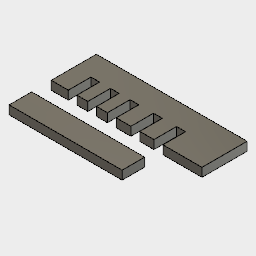
test kit with dog bone (Autodesk Fusion 360 design; units mm, degrees)
Autodesk Fusion 360 part; units mm, degrees
note: some values were not read from the file. Set by a fixed rule: which sketch regions a step uses.
sketch "Sketch1" plane through (0, 0, 0) normal (0, 1, 0) x (1, 0, 0)
  line L0 (-84.8022, -30) -> (-72.2022, -30)
  line L1 (-72.2022, -30) -> (-72.2022, 0)
  line L2 (-72.2022, 0) -> (-84.8022, 0)
  line L3 (-84.8022, 0) -> (-84.8022, -30)
  line L4 (-53.694, -30) -> (-40.994, -30)
  line L5 (-40.994, -30) -> (-40.994, 0)
  line L6 (-40.994, 0) -> (-53.694, 0)
  line L7 (-53.694, 0) -> (-53.694, -30)
  line L8 (-23.1582, -30) -> (-10.3582, -30)
  line L9 (-10.3582, -30) -> (-10.3582, 0)
  line L10 (-10.3582, 0) -> (-23.1582, 0)
  line L11 (-23.1582, 0) -> (-23.1582, -30)
  line L12 (-99.2349, -30) -> (-111.7349, -30)
  line L13 (-111.7349, -30) -> (-111.7349, 0)
  line L14 (-111.7349, 0) -> (-99.2349, 0)
  line L15 (-99.2349, 0) -> (-99.2349, -30)
  line L16 (-125.224, -30) -> (-137.624, -30)
  line L17 (-137.624, -30) -> (-137.624, 0)
  line L18 (-137.624, 0) -> (-125.224, 0)
  line L19 (-125.224, 0) -> (-125.224, -30)
  line L20 (-159.4563, -30) -> (40.5437, -30)
  line L21 (40.5437, -30) -> (40.5437, 30)
  line L22 (40.5437, 30) -> (-159.4563, 30)
  line L23 (-159.4563, 30) -> (-159.4563, -30)
  dimension "d3" = 12.6
  dimension "d4" = 30
  dimension "d6" = 12.7
  dimension "d7" = 30
  dimension "d8" = 12.8
  dimension "d9" = 30
  dimension "d10" = 12.5
  dimension "d11" = 30
  dimension "d12" = 12.4
  dimension "d13" = 30
  dimension "d14" = 200
  dimension "d15" = 60
  measures "d3" distance of L0.start L0.end
  measures "d4" distance of L0.start L2.end
  measures "d6" distance of L4.start L4.end
  measures "d7" distance of L4.start L6.end
  measures "d8" distance of L8.start L8.end
  measures "d9" distance of L8.start L10.end
  measures "d10" distance of L12.start L12.end
  measures "d11" distance of L12.start L14.end
  measures "d12" distance of L16.start L16.end
  measures "d13" distance of L16.start L18.end
  measures "d14" distance of L20.start L20.end
  measures "d15" distance of L20.start L22.end
extrude "Extrude1" add sketch "Sketch1" along normal blind 11.6 contours L1 L2 L3 L5 L6 L7 L9 L10 L11 L13 L14 L15 L17 L18 L19 L20 L21 L22 L23 makes body 1
sketch "Sketch2" plane through (0, 11.6, 0) normal (0, 1, 0) x (-1, 0, 0)
  line L0 (10.3582, 30) -> (-40.5437, 30)
  line L1 (-40.5437, 30) -> (-40.5437, -30)
  line L2 (-40.5437, -30) -> (159.4563, -30)
  line L3 (159.4563, -30) -> (159.4563, 30)
  line L4 (159.4563, 30) -> (137.624, 30)
  line L5 (137.624, 30) -> (137.624, 0)
  line L6 (137.624, 0) -> (125.224, 0)
  line L7 (125.224, 0) -> (125.224, 30)
  line L8 (125.224, 30) -> (111.7349, 30)
  line L9 (111.7349, 30) -> (111.7349, 0)
  line L10 (111.7349, 0) -> (99.2349, 0)
  line L11 (99.2349, 0) -> (99.2349, 30)
  line L12 (99.2349, 30) -> (84.8022, 30)
  line L13 (84.8022, 30) -> (84.8022, 0)
  line L14 (84.8022, 0) -> (72.2022, 0)
  line L15 (72.2022, 0) -> (72.2022, 30)
  line L16 (72.2022, 30) -> (53.694, 30)
  line L17 (53.694, 30) -> (53.694, 0)
  line L18 (53.694, 0) -> (40.994, 0)
  line L19 (40.994, 0) -> (40.994, 30)
  line L20 (40.994, 30) -> (23.1582, 30)
  line L21 (23.1582, 30) -> (23.1582, 0)
  line L22 (23.1582, 0) -> (10.3582, 0)
  line L23 (10.3582, 0) -> (10.3582, 30)
  line L24 (159.1299, 46.1552) -> (9.1299, 46.1552)
  line L25 (9.1299, 46.1552) -> (9.1299, 76.1552)
  line L26 (9.1299, 76.1552) -> (159.1299, 76.1552)
  line L27 (159.1299, 76.1552) -> (159.1299, 46.1552)
  dimension "d18" = 150
  dimension "d19" = 30
  measures "d18" distance of L24.start L24.end
  measures "d19" distance of L24.start L26.end
extrude "Extrude2" add sketch "Sketch2" along normal blind 11.6 separate body contours L24 L25 L26 L27 makes body 2
move_body "Move1" bodies 2 to x (1, 0, 0) y (0, 1, 0) z (0, 0, 1) at (0, 0, 10)
move_body "Align1" bodies 2 to x (1, 0, 0) y (0, 1, 0) z (0, 0, 1) at (0, -11.6, 0)
sketch "Sketch3" plane through (0, 0, 0) normal (0, 1, 0) x (1, 0, 0)
  line L0 (-135.0903, -41.1348) -> (-85.0903, -41.1348)
  line L1 (-85.0903, -41.1348) -> (-85.0903, -68.6348)
  line L2 (-85.0903, -68.6348) -> (-135.0903, -68.6348)
  line L3 (-135.0903, -68.6348) -> (-135.0903, -41.1348)
  dimension "d22" = 50
  dimension "d23" = 27.5
  measures "d22" distance of L0.start L0.end
  measures "d23" distance of L0.start L2.end
extrude "Extrude3" add sketch "Sketch3" along normal blind 11.6 separate body makes body 3
delete_body "RemoveBody1" bodies 2
move_body "Move2" bodies 3 to x (1, 0, 0) y (0, 1, 0) z (0, 0, 1) at (-20, 0, 20)
sketch "Sketch4" plane through (0, 11.6, 0) normal (0, 1, 0) x (-1, 0, 0)
  line L0 (10.3582, 30) -> (-40.5437, 30)
  line L1 (-40.5437, 30) -> (-40.5437, -30)
  line L2 (-40.5437, -30) -> (159.4563, -30)
  line L3 (159.4563, -30) -> (159.4563, 30)
  line L4 (159.4563, 30) -> (137.624, 30)
  line L5 (137.624, 30) -> (137.624, 0)
  line L6 (137.624, 0) -> (125.224, 0)
  line L7 (125.224, 0) -> (125.224, 30)
  line L8 (125.224, 30) -> (111.7349, 30)
  line L9 (111.7349, 30) -> (111.7349, 0)
  line L10 (111.7349, 0) -> (99.2349, 0)
  line L11 (99.2349, 0) -> (99.2349, 30)
  line L12 (99.2349, 30) -> (84.8022, 30)
  line L13 (84.8022, 30) -> (84.8022, 0)
  line L14 (84.8022, 0) -> (72.2022, 0)
  line L15 (72.2022, 0) -> (72.2022, 30)
  line L16 (72.2022, 30) -> (53.694, 30)
  line L17 (53.694, 30) -> (53.694, 0)
  line L18 (53.694, 0) -> (40.994, 0)
  line L19 (40.994, 0) -> (40.994, 30)
  line L20 (40.994, 30) -> (23.1582, 30)
  line L21 (23.1582, 30) -> (23.1582, 0)
  line L22 (23.1582, 0) -> (10.3582, 0)
  line L23 (10.3582, 0) -> (10.3582, 30)
  circle A0 centre (137.624, 0) radius 3
  circle A1 centre (125.224, 0) radius 3
  circle A2 centre (111.7349, 0) radius 3
  circle A3 centre (99.2349, 0) radius 3
  circle A4 centre (84.8022, 0) radius 3
  circle A5 centre (72.2022, 0) radius 3
  circle A6 centre (53.694, 0) radius 3
  circle A7 centre (40.994, 0) radius 3
  circle A8 centre (23.1582, 0) radius 3
  circle A9 centre (10.3582, 0) radius 3
  dimension "d27" = 6
  dimension "d28" = 6
  dimension "d29" = 6
  dimension "d30" = 6
  dimension "d31" = 6
  dimension "d32" = 6
  dimension "d33" = 6
  dimension "d34" = 6
  dimension "d35" = 6
  dimension "d36" = 6
  measures "d27" diameter of A0
  measures "d28" diameter of A1
  measures "d29" diameter of A2
  measures "d30" diameter of A3
  measures "d31" diameter of A4
  measures "d32" diameter of A5
  measures "d33" diameter of A6
  measures "d34" diameter of A7
  measures "d35" diameter of A8
  measures "d36" diameter of A9
extrude "Extrude4" cut sketch "Sketch4" against normal blind 11.6 contours L22 L23 A9 | L21 L22 A8 | L5 L6 A0 | L18 L19 A7 | L6 L7 A1 | L17 L18 A6 | L9 L10 A2 | L14 L15 A5 | L10 L11 A3 | L13 L14 A4 picked at (11.9306, -1.2271) picked at (25.1471, -0.149) picked at (139.6128, -0.149) picked at (41.0429, -1.994) picked at (126.1208, -1.7816) picked at (55.6828, -0.149) picked at (113.7238, -0.149) picked at (73.099, -1.7816) picked at (100.1317, -1.7816) picked at (82.8134, -0.149) bodies 1
equation "d3 = thickness + 1 mm"
equation "thickness = 11.6 mm"
equation "d6 = thickness + 1.1 mm"
equation "d8 = thickness + 1.2 mm"
equation "d10 = thickness + 0.9 mm"
equation "d12 = thickness + 0.8 mm"
equation "d16 = thickness"
equation "d20 = thickness"
equation "d24 = thickness"
equation "tool = 6 mm"
equation "d27 = tool"
equation "d28 = tool"
equation "d29 = tool"
equation "d30 = tool"
equation "d31 = tool"
equation "d32 = tool"
equation "d33 = tool"
equation "d34 = tool"
equation "d35 = tool"
equation "d36 = tool"
equation "d37 = -thickness"
